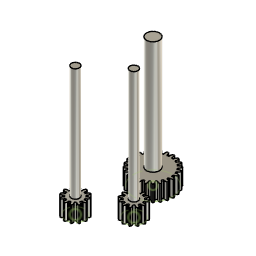
axle with gears v1 (Autodesk Fusion 360 design; units mm, degrees)
description: Spur Gear; Module: 2.000000; Num Teeth: 24; Pressure Angle: 20.000000; Backlash: 0.00 mm
description: Spur Gear; Module: 1.000000; Num Teeth: 24; Pressure Angle: 20.000000; Backlash: 0.00 mm
description: Spur Gear; Module: 0.500000; Num Teeth: 12; Pressure Angle: 20.000000; Backlash: 0.00 mm
description: Spur Gear; Module: 1.000000; Num Teeth: 12; Pressure Angle: 20.000000; Backlash: 0.00 mm
Autodesk Fusion 360 part; units mm, degrees
(part 1 of 7)
sketch "Sketch1" plane through (0, 0, 0) normal (0, 0, 1) x (1, 0, 0)
sketch "Sketch1 (2)" plane through (0, 0, 0) normal (0, 0, 1) x (1, 0, 0) in component "Spur Gear (24 teeth)"
  circle A0 centre (0, 0) radius 21.5492
extrude "Extrude1" [suppressed] in component "Spur Gear (24 teeth)"
sketch "Sketch2" plane through (0, 0, 0) normal (0, 0, 1) x (1, 0, 0) in component "Spur Gear (24 teeth)"
  spline S0 degree 5 poles (22.4799, -1.8102) (22.4899, -1.8111) (22.5101, -1.8124) (22.5404, -1.8137) (22.5808, -1.814) (22.6313, -1.8123) (22.6819, -1.8093) (22.7326, -1.8054) (22.7832, -1.801) (22.8339, -1.7962) (22.8846, -1.7911) (22.9353, -1.7856) (22.986, -1.7795) (23.0367, -1.7727) (23.0874, -1.7652) (23.1381, -1.7571) (23.1889, -1.7484) (23.2396, -1.7393) (23.2903, -1.7297) (23.341, -1.7198) (23.3916, -1.7095) (23.4423, -1.6988) (23.493, -1.6877) (23.5436, -1.6762) (23.5943, -1.6642) (23.6449, -1.6518) (23.6955, -1.6391) (23.7461, -1.6259) (23.7966, -1.6124) (23.8472, -1.5986) (23.8977, -1.5844) (23.9482, -1.5699) (23.9987, -1.555) (24.0491, -1.5398) (24.0996, -1.5242) (24.15, -1.5083) (24.2004, -1.4921) (24.2507, -1.4756) (24.301, -1.4587) (24.3513, -1.4415) (24.4016, -1.424) (24.4518, -1.4062) (24.502, -1.3881) (24.5522, -1.3697) (24.6024, -1.351) (24.6525, -1.3321) (24.7025, -1.3128) (24.7526, -1.2932) (24.8026, -1.2733) (24.8525, -1.2532) (24.9025, -1.2327) (24.9523, -1.212) (25.0022, -1.191) (25.052, -1.1697) (25.1018, -1.1482) (25.1515, -1.1264) (25.2012, -1.1043) (25.2509, -1.0819) (25.3005, -1.0593) (25.35, -1.0364) (25.3995, -1.0133) (25.449, -0.9898) (25.4985, -0.9662) (25.5478, -0.9422) (25.5972, -0.9181) (25.6465, -0.8936) (25.6957, -0.8689) (25.7449, -0.844) (25.7941, -0.8188) (25.8432, -0.7933) (25.8922, -0.7676) (25.9314, -0.7469) (25.9608, -0.7312) (25.9804, -0.7207) (25.9902, -0.7155) knots 0 0 0 0 0 0 0.01428571 0.02857143 0.04285714 0.05714286 0.07142857 0.08571429 0.1 0.11428571 0.12857143 0.14285714 0.15714286 0.17142857 0.18571429 0.2 0.21428571 0.22857143 0.24285714 0.25714286 0.27142857 0.28571429 0.3 0.31428571 0.32857143 0.34285714 0.35714286 0.37142857 0.38571429 0.4 0.41428571 0.42857143 0.44285714 0.45714286 0.47142857 0.48571429 0.5 0.51428571 0.52857143 0.54285714 0.55714286 0.57142857 0.58571429 0.6 0.61428571 0.62857143 0.64285714 0.65714286 0.67142857 0.68571429 0.7 0.71428571 0.72857143 0.74285714 0.75714286 0.77142857 0.78571429 0.8 0.81428571 0.82857143 0.84285714 0.85714286 0.87142857 0.88571429 0.9 0.91428571 0.92857143 0.94285714 0.95714286 0.97142857 0.98571429 1 1 1 1 1 1
  spline S1 degree 5 poles (22.4799, 1.8102) (22.4899, 1.8111) (22.5101, 1.8124) (22.5404, 1.8137) (22.5808, 1.814) (22.6313, 1.8123) (22.6819, 1.8093) (22.7326, 1.8054) (22.7832, 1.801) (22.8339, 1.7962) (22.8846, 1.7911) (22.9353, 1.7856) (22.986, 1.7795) (23.0367, 1.7727) (23.0874, 1.7652) (23.1381, 1.7571) (23.1889, 1.7484) (23.2396, 1.7393) (23.2903, 1.7297) (23.341, 1.7198) (23.3916, 1.7095) (23.4423, 1.6988) (23.493, 1.6877) (23.5436, 1.6762) (23.5943, 1.6642) (23.6449, 1.6518) (23.6955, 1.6391) (23.7461, 1.6259) (23.7966, 1.6124) (23.8472, 1.5986) (23.8977, 1.5844) (23.9482, 1.5699) (23.9987, 1.555) (24.0491, 1.5398) (24.0996, 1.5242) (24.15, 1.5083) (24.2004, 1.4921) (24.2507, 1.4756) (24.301, 1.4587) (24.3513, 1.4415) (24.4016, 1.424) (24.4518, 1.4062) (24.502, 1.3881) (24.5522, 1.3697) (24.6024, 1.351) (24.6525, 1.3321) (24.7025, 1.3128) (24.7526, 1.2932) (24.8026, 1.2733) (24.8525, 1.2532) (24.9025, 1.2327) (24.9523, 1.212) (25.0022, 1.191) (25.052, 1.1697) (25.1018, 1.1482) (25.1515, 1.1264) (25.2012, 1.1043) (25.2509, 1.0819) (25.3005, 1.0593) (25.35, 1.0364) (25.3995, 1.0133) (25.449, 0.9898) (25.4985, 0.9662) (25.5478, 0.9422) (25.5972, 0.9181) (25.6465, 0.8936) (25.6957, 0.8689) (25.7449, 0.844) (25.7941, 0.8188) (25.8432, 0.7933) (25.8922, 0.7676) (25.9314, 0.7469) (25.9608, 0.7312) (25.9804, 0.7207) (25.9902, 0.7155) knots 0 0 0 0 0 0 0.01428571 0.02857143 0.04285714 0.05714286 0.07142857 0.08571429 0.1 0.11428571 0.12857143 0.14285714 0.15714286 0.17142857 0.18571429 0.2 0.21428571 0.22857143 0.24285714 0.25714286 0.27142857 0.28571429 0.3 0.31428571 0.32857143 0.34285714 0.35714286 0.37142857 0.38571429 0.4 0.41428571 0.42857143 0.44285714 0.45714286 0.47142857 0.48571429 0.5 0.51428571 0.52857143 0.54285714 0.55714286 0.57142857 0.58571429 0.6 0.61428571 0.62857143 0.64285714 0.65714286 0.67142857 0.68571429 0.7 0.71428571 0.72857143 0.74285714 0.75714286 0.77142857 0.78571429 0.8 0.81428571 0.82857143 0.84285714 0.85714286 0.87142857 0.88571429 0.9 0.91428571 0.92857143 0.94285714 0.95714286 0.97142857 0.98571429 1 1 1 1 1 1
  arc A0 (25.9902, -0.7155) -> (25.9902, 0.7155) centre (0, 0) ccw
  line L0 (21.4697, -1.7297) -> (22.4799, -1.8102)
  line L1 (21.4697, 1.7297) -> (22.4799, 1.8102)
  line L2 (21.4697, -1.7297) -> (21.4697, 1.7297)
  point P0 (22.7272, -1.8057)
  point P1 (22.9762, -1.7806)
  point P2 (23.2261, -1.7416)
  point P3 (23.4768, -1.6912)
  point P4 (23.7279, -1.6306)
  point P5 (23.9793, -1.5607)
  point P6 (24.231, -1.482)
  point P7 (24.4828, -1.395)
  point P8 (24.7346, -1.3002)
  point P9 (24.9863, -1.1976)
  point P10 (25.2378, -1.0877)
  point P11 (25.489, -0.9706)
  point P12 (25.7398, -0.8465)
  point P13 (22.7272, 1.8057)
  point P14 (22.9762, 1.7806)
  point P15 (23.2261, 1.7416)
  point P16 (23.4768, 1.6912)
  point P17 (23.7279, 1.6306)
  point P18 (23.9793, 1.5607)
  point P19 (24.231, 1.482)
  point P20 (24.4828, 1.395)
  point P21 (24.7346, 1.3002)
  point P22 (24.9863, 1.1976)
  point P23 (25.2378, 1.0877)
  point P24 (25.489, 0.9706)
  point P25 (25.7398, 0.8465)
extrude "Extrude2" [suppressed] in component "Spur Gear (24 teeth)"
pattern_circular "C-Pattern1" [suppressed] in component "Spur Gear (24 teeth)"
sketch "Sketch3" plane through (0, 0, 0) normal (0, 0, 1) x (1, 0, 0) in component "Spur Gear (24 teeth)"
  circle A0 centre (0, 0) radius 24 construction
sketch "Sketch1 (3)" plane through (0, 0, 0) normal (0, 0, 1) x (1, 0, 0) in component "Spur Gear (24 teeth) (1)"
  circle A0 centre (0, 0) radius 10.7492
extrude "Extrude1'" add sketch "Sketch1 (3)" along normal blind 10 makes body 1 in component "Spur Gear (24 teeth) (1)"
sketch "Sketch2 (2)" plane through (0, 0, 0) normal (0, 0, 1) x (1, 0, 0) in component "Spur Gear (24 teeth) (1)"
  spline S0 degree 5 poles (11.2399, -0.9051) (11.2449, -0.9055) (11.255, -0.9062) (11.27, -0.9068) (11.2901, -0.907) (11.3152, -0.9062) (11.3404, -0.9047) (11.3655, -0.9028) (11.3907, -0.9006) (11.416, -0.8982) (11.4412, -0.8957) (11.4664, -0.8929) (11.4917, -0.8899) (11.5169, -0.8866) (11.5422, -0.8828) (11.5674, -0.8788) (11.5927, -0.8745) (11.6179, -0.87) (11.6432, -0.8652) (11.6685, -0.8603) (11.6937, -0.8552) (11.719, -0.8499) (11.7443, -0.8443) (11.7695, -0.8386) (11.7948, -0.8327) (11.82, -0.8265) (11.8453, -0.8202) (11.8706, -0.8136) (11.8958, -0.8069) (11.921, -0.8) (11.9463, -0.7929) (11.9715, -0.7857) (11.9967, -0.7783) (12.0219, -0.7707) (12.0471, -0.7629) (12.0723, -0.755) (12.0975, -0.7469) (12.1227, -0.7387) (12.1479, -0.7302) (12.173, -0.7217) (12.1982, -0.7129) (12.2233, -0.7041) (12.2484, -0.695) (12.2735, -0.6858) (12.2986, -0.6765) (12.3237, -0.667) (12.3488, -0.6573) (12.3739, -0.6475) (12.3989, -0.6376) (12.424, -0.6275) (12.449, -0.6173) (12.474, -0.6069) (12.499, -0.5964) (12.5239, -0.5858) (12.5489, -0.575) (12.5738, -0.564) (12.5988, -0.553) (12.6237, -0.5418) (12.6486, -0.5304) (12.6735, -0.5189) (12.6983, -0.5073) (12.7232, -0.4956) (12.748, -0.4837) (12.7728, -0.4717) (12.7976, -0.4595) (12.8223, -0.4473) (12.8471, -0.4349) (12.8718, -0.4223) (12.8965, -0.4097) (12.9212, -0.3969) (12.9458, -0.384) (12.9655, -0.3735) (12.9803, -0.3657) (12.9902, -0.3604) (12.9951, -0.3577) knots 0 0 0 0 0 0 0.01428571 0.02857143 0.04285714 0.05714286 0.07142857 0.08571429 0.1 0.11428571 0.12857143 0.14285714 0.15714286 0.17142857 0.18571429 0.2 0.21428571 0.22857143 0.24285714 0.25714286 0.27142857 0.28571429 0.3 0.31428571 0.32857143 0.34285714 0.35714286 0.37142857 0.38571429 0.4 0.41428571 0.42857143 0.44285714 0.45714286 0.47142857 0.48571429 0.5 0.51428571 0.52857143 0.54285714 0.55714286 0.57142857 0.58571429 0.6 0.61428571 0.62857143 0.64285714 0.65714286 0.67142857 0.68571429 0.7 0.71428571 0.72857143 0.74285714 0.75714286 0.77142857 0.78571429 0.8 0.81428571 0.82857143 0.84285714 0.85714286 0.87142857 0.88571429 0.9 0.91428571 0.92857143 0.94285714 0.95714286 0.97142857 0.98571429 1 1 1 1 1 1
  spline S1 degree 5 poles (11.2399, 0.9051) (11.2449, 0.9055) (11.255, 0.9062) (11.27, 0.9068) (11.2901, 0.907) (11.3152, 0.9062) (11.3404, 0.9047) (11.3655, 0.9028) (11.3907, 0.9006) (11.416, 0.8982) (11.4412, 0.8957) (11.4664, 0.8929) (11.4917, 0.8899) (11.5169, 0.8866) (11.5422, 0.8828) (11.5674, 0.8788) (11.5927, 0.8745) (11.6179, 0.87) (11.6432, 0.8652) (11.6685, 0.8603) (11.6937, 0.8552) (11.719, 0.8499) (11.7443, 0.8443) (11.7695, 0.8386) (11.7948, 0.8327) (11.82, 0.8265) (11.8453, 0.8202) (11.8706, 0.8136) (11.8958, 0.8069) (11.921, 0.8) (11.9463, 0.7929) (11.9715, 0.7857) (11.9967, 0.7783) (12.0219, 0.7707) (12.0471, 0.7629) (12.0723, 0.755) (12.0975, 0.7469) (12.1227, 0.7387) (12.1479, 0.7302) (12.173, 0.7217) (12.1982, 0.7129) (12.2233, 0.7041) (12.2484, 0.695) (12.2735, 0.6858) (12.2986, 0.6765) (12.3237, 0.667) (12.3488, 0.6573) (12.3739, 0.6475) (12.3989, 0.6376) (12.424, 0.6275) (12.449, 0.6173) (12.474, 0.6069) (12.499, 0.5964) (12.5239, 0.5858) (12.5489, 0.575) (12.5738, 0.564) (12.5988, 0.553) (12.6237, 0.5418) (12.6486, 0.5304) (12.6735, 0.5189) (12.6983, 0.5073) (12.7232, 0.4956) (12.748, 0.4837) (12.7728, 0.4717) (12.7976, 0.4595) (12.8223, 0.4473) (12.8471, 0.4349) (12.8718, 0.4223) (12.8965, 0.4097) (12.9212, 0.3969) (12.9458, 0.384) (12.9655, 0.3735) (12.9803, 0.3657) (12.9902, 0.3604) (12.9951, 0.3577) knots 0 0 0 0 0 0 0.01428571 0.02857143 0.04285714 0.05714286 0.07142857 0.08571429 0.1 0.11428571 0.12857143 0.14285714 0.15714286 0.17142857 0.18571429 0.2 0.21428571 0.22857143 0.24285714 0.25714286 0.27142857 0.28571429 0.3 0.31428571 0.32857143 0.34285714 0.35714286 0.37142857 0.38571429 0.4 0.41428571 0.42857143 0.44285714 0.45714286 0.47142857 0.48571429 0.5 0.51428571 0.52857143 0.54285714 0.55714286 0.57142857 0.58571429 0.6 0.61428571 0.62857143 0.64285714 0.65714286 0.67142857 0.68571429 0.7 0.71428571 0.72857143 0.74285714 0.75714286 0.77142857 0.78571429 0.8 0.81428571 0.82857143 0.84285714 0.85714286 0.87142857 0.88571429 0.9 0.91428571 0.92857143 0.94285714 0.95714286 0.97142857 0.98571429 1 1 1 1 1 1
  arc A0 (12.9951, -0.3577) -> (12.9951, 0.3577) centre (0, 0) ccw
  line L0 (10.7045, -0.8628) -> (11.2399, -0.9051)
  line L1 (10.7045, 0.8628) -> (11.2399, 0.9051)
  line L2 (10.7045, -0.8628) -> (10.7045, 0.8628)
  point P0 (11.3636, -0.9028)
  point P1 (11.4881, -0.8903)
  point P2 (11.6131, -0.8708)
  point P3 (11.7384, -0.8456)
  point P4 (11.8639, -0.8153)
  point P5 (11.9897, -0.7803)
  point P6 (12.1155, -0.741)
  point P7 (12.2414, -0.6975)
  point P8 (12.3673, -0.6501)
  point P9 (12.4932, -0.5988)
  point P10 (12.6189, -0.5439)
  point P11 (12.7445, -0.4853)
  point P12 (12.8699, -0.4232)
  point P13 (11.3636, 0.9028)
  point P14 (11.4881, 0.8903)
  point P15 (11.6131, 0.8708)
  point P16 (11.7384, 0.8456)
  point P17 (11.8639, 0.8153)
  point P18 (11.9897, 0.7803)
  point P19 (12.1155, 0.741)
  point P20 (12.2414, 0.6975)
  point P21 (12.3673, 0.6501)
  point P22 (12.4932, 0.5988)
  point P23 (12.6189, 0.5439)
  point P24 (12.7445, 0.4853)
  point P25 (12.8699, 0.4232)
extrude "Extrude2'" add sketch "Sketch2 (2)" along normal blind 10 bodies 1 in component "Spur Gear (24 teeth) (1)"
pattern_circular "C-Pattern1'" count 24 over 360 about axis through (0, 0, 0) along (0, 0, 1) of "Extrude2'" in component "Spur Gear (24 teeth) (1)"
sketch "Sketch3 (2)" plane through (0, 0, 0) normal (0, 0, 1) x (1, 0, 0) in component "Spur Gear (24 teeth) (1)"
  circle A0 centre (0, 0) radius 12 construction
sketch "Sketch2 (3)" plane through (0, 0, 0) normal (0, 0, -1) x (1, 0, 0)
  arc A0 (10.1259, 3.6073) -> (9.7108, 4.6093) centre (0, 0) ccw
  line L0 (9.7108, 4.6093) -> (10.1866, 4.8361)
  spline S0 degree 5 poles (10.1866, 4.8361) (10.1912, 4.8383) (10.2002, 4.8427) (10.2135, 4.8497) (10.231, 4.8596) (10.2523, 4.8728) (10.2734, 4.8867) (10.2942, 4.901) (10.315, 4.9155) (10.3356, 4.9301) (10.3562, 4.9449) (10.3767, 4.9599) (10.397, 4.9751) (10.4172, 4.9907) (10.4372, 5.0065) (10.4571, 5.0226) (10.4768, 5.039) (10.4964, 5.0555) (10.5159, 5.0723) (10.5353, 5.0892) (10.5547, 5.1063) (10.5739, 5.1235) (10.593, 5.1409) (10.612, 5.1585) (10.6309, 5.1763) (10.6497, 5.1942) (10.6684, 5.2124) (10.687, 5.2307) (10.7055, 5.2491) (10.7239, 5.2677) (10.7422, 5.2864) (10.7605, 5.3053) (10.7786, 5.3243) (10.7966, 5.3435) (10.8146, 5.3628) (10.8324, 5.3823) (10.8502, 5.4019) (10.8679, 5.4216) (10.8855, 5.4415) (10.903, 5.4615) (10.9204, 5.4817) (10.9377, 5.5019) (10.955, 5.5223) (10.9721, 5.5428) (10.9892, 5.5635) (11.0062, 5.5842) (11.023, 5.6051) (11.0399, 5.6261) (11.0566, 5.6473) (11.0732, 5.6685) (11.0898, 5.6899) (11.1062, 5.7114) (11.1226, 5.733) (11.1389, 5.7547) (11.1552, 5.7765) (11.1713, 5.7985) (11.1873, 5.8205) (11.2033, 5.8427) (11.2192, 5.8649) (11.235, 5.8873) (11.2507, 5.9098) (11.2664, 5.9324) (11.2819, 5.9551) (11.2974, 5.9779) (11.3128, 6.0008) (11.3281, 6.0238) (11.3433, 6.0469) (11.3585, 6.0701) (11.3735, 6.0935) (11.3885, 6.1169) (11.4034, 6.1404) (11.4153, 6.1593) (11.4241, 6.1735) (11.43, 6.183) (11.4329, 6.1877) knots 0 0 0 0 0 0 0.01428571 0.02857143 0.04285714 0.05714286 0.07142857 0.08571429 0.1 0.11428571 0.12857143 0.14285714 0.15714286 0.17142857 0.18571429 0.2 0.21428571 0.22857143 0.24285714 0.25714286 0.27142857 0.28571429 0.3 0.31428571 0.32857143 0.34285714 0.35714286 0.37142857 0.38571429 0.4 0.41428571 0.42857143 0.44285714 0.45714286 0.47142857 0.48571429 0.5 0.51428571 0.52857143 0.54285714 0.55714286 0.57142857 0.58571429 0.6 0.61428571 0.62857143 0.64285714 0.65714286 0.67142857 0.68571429 0.7 0.71428571 0.72857143 0.74285714 0.75714286 0.77142857 0.78571429 0.8 0.81428571 0.82857143 0.84285714 0.85714286 0.87142857 0.88571429 0.9 0.91428571 0.92857143 0.94285714 0.95714286 0.97142857 0.98571429 1 1 1 1 1 1
  arc A1 (11.4329, 6.1877) -> (11.0752, 6.8073) centre (0, 0) ccw
  spline S1 degree 5 poles (9.2815, 6.4038) (9.2856, 6.4067) (9.294, 6.4123) (9.3067, 6.4203) (9.324, 6.4305) (9.3462, 6.4424) (9.3687, 6.4537) (9.3915, 6.4646) (9.4144, 6.4753) (9.4374, 6.4859) (9.4605, 6.4963) (9.4837, 6.5065) (9.5071, 6.5165) (9.5307, 6.5262) (9.5544, 6.5356) (9.5783, 6.5448) (9.6023, 6.5537) (9.6264, 6.5624) (9.6507, 6.5709) (9.675, 6.5793) (9.6995, 6.5875) (9.724, 6.5955) (9.7487, 6.6034) (9.7734, 6.611) (9.7983, 6.6185) (9.8232, 6.6258) (9.8483, 6.6329) (9.8734, 6.6399) (9.8986, 6.6467) (9.9239, 6.6533) (9.9493, 6.6598) (9.9748, 6.6662) (10.0003, 6.6724) (10.0259, 6.6784) (10.0516, 6.6843) (10.0774, 6.69) (10.1033, 6.6956) (10.1292, 6.701) (10.1552, 6.7063) (10.1813, 6.7115) (10.2074, 6.7165) (10.2337, 6.7214) (10.2599, 6.7261) (10.2863, 6.7307) (10.3127, 6.7352) (10.3392, 6.7395) (10.3657, 6.7437) (10.3923, 6.7477) (10.419, 6.7516) (10.4457, 6.7554) (10.4725, 6.7591) (10.4993, 6.7626) (10.5262, 6.766) (10.5532, 6.7693) (10.5802, 6.7724) (10.6073, 6.7754) (10.6344, 6.7783) (10.6616, 6.781) (10.6888, 6.7836) (10.7161, 6.7861) (10.7434, 6.7885) (10.7708, 6.7908) (10.7982, 6.7929) (10.8257, 6.7949) (10.8532, 6.7967) (10.8808, 6.7985) (10.9085, 6.8001) (10.9361, 6.8016) (10.9638, 6.803) (10.9916, 6.8043) (11.0194, 6.8054) (11.0417, 6.8063) (11.0585, 6.8068) (11.0696, 6.8072) (11.0752, 6.8073) knots 0 0 0 0 0 0 0.01428571 0.02857143 0.04285714 0.05714286 0.07142857 0.08571429 0.1 0.11428571 0.12857143 0.14285714 0.15714286 0.17142857 0.18571429 0.2 0.21428571 0.22857143 0.24285714 0.25714286 0.27142857 0.28571429 0.3 0.31428571 0.32857143 0.34285714 0.35714286 0.37142857 0.38571429 0.4 0.41428571 0.42857143 0.44285714 0.45714286 0.47142857 0.48571429 0.5 0.51428571 0.52857143 0.54285714 0.55714286 0.57142857 0.58571429 0.6 0.61428571 0.62857143 0.64285714 0.65714286 0.67142857 0.68571429 0.7 0.71428571 0.72857143 0.74285714 0.75714286 0.77142857 0.78571429 0.8 0.81428571 0.82857143 0.84285714 0.85714286 0.87142857 0.88571429 0.9 0.91428571 0.92857143 0.94285714 0.95714286 0.97142857 0.98571429 1 1 1 1 1 1
  line L1 (9.2815, 6.4038) -> (8.8472, 6.1051)
  arc A2 (8.8472, 6.1051) -> (8.1869, 6.9656) centre (0, 0) ccw
  line L2 (8.1869, 6.9656) -> (8.5878, 7.3078)
  spline S2 degree 5 poles (8.5878, 7.3078) (8.5917, 7.3111) (8.5992, 7.3177) (8.6103, 7.3279) (8.6246, 7.342) (8.6418, 7.3603) (8.6586, 7.3791) (8.675, 7.3983) (8.6913, 7.4177) (8.7074, 7.4372) (8.7235, 7.4568) (8.7394, 7.4766) (8.7551, 7.4966) (8.7706, 7.5168) (8.7858, 7.5373) (8.8008, 7.558) (8.8156, 7.5789) (8.8303, 7.6) (8.8448, 7.6212) (8.8592, 7.6425) (8.8734, 7.664) (8.8875, 7.6856) (8.9015, 7.7074) (8.9153, 7.7293) (8.929, 7.7514) (8.9425, 7.7736) (8.9558, 7.796) (8.9691, 7.8184) (8.9822, 7.841) (8.9951, 7.8638) (9.008, 7.8866) (9.0207, 7.9096) (9.0333, 7.9326) (9.0457, 7.9558) (9.0581, 7.9791) (9.0703, 8.0025) (9.0824, 8.0261) (9.0943, 8.0497) (9.1062, 8.0735) (9.1179, 8.0973) (9.1295, 8.1213) (9.141, 8.1453) (9.1524, 8.1695) (9.1637, 8.1938) (9.1748, 8.2181) (9.1858, 8.2426) (9.1967, 8.2671) (9.2075, 8.2918) (9.2182, 8.3165) (9.2288, 8.3413) (9.2392, 8.3663) (9.2496, 8.3913) (9.2598, 8.4164) (9.27, 8.4416) (9.28, 8.4669) (9.2899, 8.4922) (9.2997, 8.5177) (9.3094, 8.5432) (9.319, 8.5688) (9.3284, 8.5945) (9.3378, 8.6203) (9.347, 8.6462) (9.3562, 8.6722) (9.3652, 8.6982) (9.3742, 8.7243) (9.383, 8.7505) (9.3917, 8.7768) (9.4004, 8.8031) (9.4089, 8.8295) (9.4173, 8.856) (9.4256, 8.8826) (9.4321, 8.9039) (9.437, 8.9199) (9.4403, 8.9306) (9.4419, 8.936) knots 0 0 0 0 0 0 0.01428571 0.02857143 0.04285714 0.05714286 0.07142857 0.08571429 0.1 0.11428571 0.12857143 0.14285714 0.15714286 0.17142857 0.18571429 0.2 0.21428571 0.22857143 0.24285714 0.25714286 0.27142857 0.28571429 0.3 0.31428571 0.32857143 0.34285714 0.35714286 0.37142857 0.38571429 0.4 0.41428571 0.42857143 0.44285714 0.45714286 0.47142857 0.48571429 0.5 0.51428571 0.52857143 0.54285714 0.55714286 0.57142857 0.58571429 0.6 0.61428571 0.62857143 0.64285714 0.65714286 0.67142857 0.68571429 0.7 0.71428571 0.72857143 0.74285714 0.75714286 0.77142857 0.78571429 0.8 0.81428571 0.82857143 0.84285714 0.85714286 0.87142857 0.88571429 0.9 0.91428571 0.92857143 0.94285714 0.95714286 0.97142857 0.98571429 1 1 1 1 1 1
  arc A3 (9.4419, 8.936) -> (8.936, 9.4419) centre (0, 0) ccw
  spline S3 degree 5 poles (7.3078, 8.5878) (7.3111, 8.5917) (7.3177, 8.5992) (7.3279, 8.6103) (7.342, 8.6246) (7.3603, 8.6418) (7.3791, 8.6586) (7.3983, 8.675) (7.4177, 8.6913) (7.4372, 8.7074) (7.4568, 8.7235) (7.4766, 8.7394) (7.4966, 8.7551) (7.5168, 8.7706) (7.5373, 8.7858) (7.558, 8.8008) (7.5789, 8.8156) (7.6, 8.8303) (7.6212, 8.8448) (7.6425, 8.8592) (7.664, 8.8734) (7.6856, 8.8875) (7.7074, 8.9015) (7.7293, 8.9153) (7.7514, 8.929) (7.7736, 8.9425) (7.796, 8.9558) (7.8184, 8.9691) (7.841, 8.9822) (7.8638, 8.9951) (7.8866, 9.008) (7.9096, 9.0207) (7.9326, 9.0333) (7.9558, 9.0457) (7.9791, 9.0581) (8.0025, 9.0703) (8.0261, 9.0824) (8.0497, 9.0943) (8.0735, 9.1062) (8.0973, 9.1179) (8.1213, 9.1295) (8.1453, 9.141) (8.1695, 9.1524) (8.1938, 9.1637) (8.2181, 9.1748) (8.2426, 9.1858) (8.2671, 9.1967) (8.2918, 9.2075) (8.3165, 9.2182) (8.3413, 9.2288) (8.3663, 9.2392) (8.3913, 9.2496) (8.4164, 9.2598) (8.4416, 9.27) (8.4669, 9.28) (8.4922, 9.2899) (8.5177, 9.2997) (8.5432, 9.3094) (8.5688, 9.319) (8.5945, 9.3284) (8.6203, 9.3378) (8.6462, 9.347) (8.6722, 9.3562) (8.6982, 9.3652) (8.7243, 9.3742) (8.7505, 9.383) (8.7768, 9.3917) (8.8031, 9.4004) (8.8295, 9.4089) (8.856, 9.4173) (8.8826, 9.4256) (8.9039, 9.4321) (8.9199, 9.437) (8.9306, 9.4403) (8.936, 9.4419) knots 0 0 0 0 0 0 0.01428571 0.02857143 0.04285714 0.05714286 0.07142857 0.08571429 0.1 0.11428571 0.12857143 0.14285714 0.15714286 0.17142857 0.18571429 0.2 0.21428571 0.22857143 0.24285714 0.25714286 0.27142857 0.28571429 0.3 0.31428571 0.32857143 0.34285714 0.35714286 0.37142857 0.38571429 0.4 0.41428571 0.42857143 0.44285714 0.45714286 0.47142857 0.48571429 0.5 0.51428571 0.52857143 0.54285714 0.55714286 0.57142857 0.58571429 0.6 0.61428571 0.62857143 0.64285714 0.65714286 0.67142857 0.68571429 0.7 0.71428571 0.72857143 0.74285714 0.75714286 0.77142857 0.78571429 0.8 0.81428571 0.82857143 0.84285714 0.85714286 0.87142857 0.88571429 0.9 0.91428571 0.92857143 0.94285714 0.95714286 0.97142857 0.98571429 1 1 1 1 1 1
  line L3 (7.3078, 8.5878) -> (6.9656, 8.1869)
  arc A4 (6.9656, 8.1869) -> (6.1051, 8.8472) centre (0, 0) ccw
  line L4 (6.1051, 8.8472) -> (6.4038, 9.2815)
  spline S4 degree 5 poles (6.4038, 9.2815) (6.4067, 9.2856) (6.4123, 9.294) (6.4203, 9.3067) (6.4305, 9.324) (6.4424, 9.3462) (6.4537, 9.3687) (6.4646, 9.3915) (6.4753, 9.4144) (6.4859, 9.4374) (6.4963, 9.4605) (6.5065, 9.4837) (6.5165, 9.5071) (6.5262, 9.5307) (6.5356, 9.5544) (6.5448, 9.5783) (6.5537, 9.6023) (6.5624, 9.6264) (6.5709, 9.6507) (6.5793, 9.675) (6.5875, 9.6995) (6.5955, 9.724) (6.6034, 9.7487) (6.611, 9.7734) (6.6185, 9.7983) (6.6258, 9.8232) (6.6329, 9.8483) (6.6399, 9.8734) (6.6467, 9.8986) (6.6533, 9.9239) (6.6598, 9.9493) (6.6662, 9.9748) (6.6724, 10.0003) (6.6784, 10.0259) (6.6843, 10.0516) (6.69, 10.0774) (6.6956, 10.1033) (6.701, 10.1292) (6.7063, 10.1552) (6.7115, 10.1813) (6.7165, 10.2074) (6.7214, 10.2337) (6.7261, 10.2599) (6.7307, 10.2863) (6.7352, 10.3127) (6.7395, 10.3392) (6.7437, 10.3657) (6.7477, 10.3923) (6.7516, 10.419) (6.7554, 10.4457) (6.7591, 10.4725) (6.7626, 10.4993) (6.766, 10.5262) (6.7693, 10.5532) (6.7724, 10.5802) (6.7754, 10.6073) (6.7783, 10.6344) (6.781, 10.6616) (6.7836, 10.6888) (6.7861, 10.7161) (6.7885, 10.7434) (6.7908, 10.7708) (6.7929, 10.7982) (6.7949, 10.8257) (6.7967, 10.8532) (6.7985, 10.8808) (6.8001, 10.9085) (6.8016, 10.9361) (6.803, 10.9638) (6.8043, 10.9916) (6.8054, 11.0194) (6.8063, 11.0417) (6.8068, 11.0585) (6.8072, 11.0696) (6.8073, 11.0752) knots 0 0 0 0 0 0 0.01428571 0.02857143 0.04285714 0.05714286 0.07142857 0.08571429 0.1 0.11428571 0.12857143 0.14285714 0.15714286 0.17142857 0.18571429 0.2 0.21428571 0.22857143 0.24285714 0.25714286 0.27142857 0.28571429 0.3 0.31428571 0.32857143 0.34285714 0.35714286 0.37142857 0.38571429 0.4 0.41428571 0.42857143 0.44285714 0.45714286 0.47142857 0.48571429 0.5 0.51428571 0.52857143 0.54285714 0.55714286 0.57142857 0.58571429 0.6 0.61428571 0.62857143 0.64285714 0.65714286 0.67142857 0.68571429 0.7 0.71428571 0.72857143 0.74285714 0.75714286 0.77142857 0.78571429 0.8 0.81428571 0.82857143 0.84285714 0.85714286 0.87142857 0.88571429 0.9 0.91428571 0.92857143 0.94285714 0.95714286 0.97142857 0.98571429 1 1 1 1 1 1
  arc A5 (6.8073, 11.0752) -> (6.1877, 11.4329) centre (0, 0) ccw
  spline S5 degree 5 poles (4.8361, 10.1866) (4.8383, 10.1912) (4.8427, 10.2002) (4.8497, 10.2135) (4.8596, 10.231) (4.8728, 10.2523) (4.8867, 10.2734) (4.901, 10.2942) (4.9155, 10.315) (4.9301, 10.3356) (4.9449, 10.3562) (4.9599, 10.3767) (4.9751, 10.397) (4.9907, 10.4172) (5.0065, 10.4372) (5.0226, 10.4571) (5.039, 10.4768) (5.0555, 10.4964) (5.0723, 10.5159) (5.0892, 10.5353) (5.1063, 10.5547) (5.1235, 10.5739) (5.1409, 10.593) (5.1585, 10.612) (5.1763, 10.6309) (5.1942, 10.6497) (5.2124, 10.6684) (5.2307, 10.687) (5.2491, 10.7055) (5.2677, 10.7239) (5.2864, 10.7422) (5.3053, 10.7605) (5.3243, 10.7786) (5.3435, 10.7966) (5.3628, 10.8146) (5.3823, 10.8324) (5.4019, 10.8502) (5.4216, 10.8679) (5.4415, 10.8855) (5.4615, 10.903) (5.4817, 10.9204) (5.5019, 10.9377) (5.5223, 10.955) (5.5428, 10.9721) (5.5635, 10.9892) (5.5842, 11.0062) (5.6051, 11.023) (5.6261, 11.0399) (5.6473, 11.0566) (5.6685, 11.0732) (5.6899, 11.0898) (5.7114, 11.1062) (5.733, 11.1226) (5.7547, 11.1389) (5.7765, 11.1552) (5.7985, 11.1713) (5.8205, 11.1873) (5.8427, 11.2033) (5.8649, 11.2192) (5.8873, 11.235) (5.9098, 11.2507) (5.9324, 11.2664) (5.9551, 11.2819) (5.9779, 11.2974) (6.0008, 11.3128) (6.0238, 11.3281) (6.0469, 11.3433) (6.0701, 11.3585) (6.0935, 11.3735) (6.1169, 11.3885) (6.1404, 11.4034) (6.1593, 11.4153) (6.1735, 11.4241) (6.183, 11.43) (6.1877, 11.4329) knots 0 0 0 0 0 0 0.01428571 0.02857143 0.04285714 0.05714286 0.07142857 0.08571429 0.1 0.11428571 0.12857143 0.14285714 0.15714286 0.17142857 0.18571429 0.2 0.21428571 0.22857143 0.24285714 0.25714286 0.27142857 0.28571429 0.3 0.31428571 0.32857143 0.34285714 0.35714286 0.37142857 0.38571429 0.4 0.41428571 0.42857143 0.44285714 0.45714286 0.47142857 0.48571429 0.5 0.51428571 0.52857143 0.54285714 0.55714286 0.57142857 0.58571429 0.6 0.61428571 0.62857143 0.64285714 0.65714286 0.67142857 0.68571429 0.7 0.71428571 0.72857143 0.74285714 0.75714286 0.77142857 0.78571429 0.8 0.81428571 0.82857143 0.84285714 0.85714286 0.87142857 0.88571429 0.9 0.91428571 0.92857143 0.94285714 0.95714286 0.97142857 0.98571429 1 1 1 1 1 1
  line L5 (4.8361, 10.1866) -> (4.6093, 9.7108)
  arc A6 (4.6093, 9.7108) -> (3.6073, 10.1259) centre (0, 0) ccw
  line L6 (3.6073, 10.1259) -> (3.7834, 10.6227)
  spline S6 degree 5 poles (3.7834, 10.6227) (3.7851, 10.6274) (3.7883, 10.6369) (3.7928, 10.6513) (3.7981, 10.6706) (3.8039, 10.6951) (3.809, 10.7198) (3.8136, 10.7446) (3.818, 10.7695) (3.8223, 10.7945) (3.8264, 10.8195) (3.8302, 10.8446) (3.8339, 10.8698) (3.8371, 10.895) (3.8401, 10.9204) (3.8427, 10.9458) (3.8451, 10.9713) (3.8473, 10.9969) (3.8492, 11.0225) (3.851, 11.0482) (3.8526, 11.0739) (3.854, 11.0997) (3.8552, 11.1256) (3.8562, 11.1514) (3.857, 11.1774) (3.8576, 11.2034) (3.858, 11.2294) (3.8582, 11.2555) (3.8583, 11.2816) (3.8581, 11.3078) (3.8578, 11.334) (3.8574, 11.3602) (3.8567, 11.3865) (3.8559, 11.4128) (3.855, 11.4392) (3.8538, 11.4656) (3.8525, 11.492) (3.8511, 11.5184) (3.8495, 11.5449) (3.8477, 11.5714) (3.8458, 11.598) (3.8437, 11.6246) (3.8415, 11.6512) (3.8391, 11.6778) (3.8365, 11.7045) (3.8339, 11.7312) (3.831, 11.7579) (3.8281, 11.7846) (3.825, 11.8114) (3.8217, 11.8382) (3.8183, 11.865) (3.8147, 11.8919) (3.8111, 11.9187) (3.8072, 11.9456) (3.8033, 11.9725) (3.7992, 11.9994) (3.7949, 12.0264) (3.7905, 12.0533) (3.786, 12.0803) (3.7814, 12.1073) (3.7766, 12.1343) (3.7717, 12.1614) (3.7666, 12.1884) (3.7614, 12.2155) (3.7561, 12.2426) (3.7507, 12.2696) (3.7451, 12.2968) (3.7394, 12.3239) (3.7336, 12.351) (3.7276, 12.3782) (3.7215, 12.4053) (3.7165, 12.4271) (3.7127, 12.4434) (3.7102, 12.4543) (3.7089, 12.4597) knots 0 0 0 0 0 0 0.01428571 0.02857143 0.04285714 0.05714286 0.07142857 0.08571429 0.1 0.11428571 0.12857143 0.14285714 0.15714286 0.17142857 0.18571429 0.2 0.21428571 0.22857143 0.24285714 0.25714286 0.27142857 0.28571429 0.3 0.31428571 0.32857143 0.34285714 0.35714286 0.37142857 0.38571429 0.4 0.41428571 0.42857143 0.44285714 0.45714286 0.47142857 0.48571429 0.5 0.51428571 0.52857143 0.54285714 0.55714286 0.57142857 0.58571429 0.6 0.61428571 0.62857143 0.64285714 0.65714286 0.67142857 0.68571429 0.7 0.71428571 0.72857143 0.74285714 0.75714286 0.77142857 0.78571429 0.8 0.81428571 0.82857143 0.84285714 0.85714286 0.87142857 0.88571429 0.9 0.91428571 0.92857143 0.94285714 0.95714286 0.97142857 0.98571429 1 1 1 1 1 1
  arc A7 (3.7089, 12.4597) -> (3.0178, 12.6449) centre (0, 0) ccw
  spline S7 degree 5 poles (2.0348, 11.0912) (2.0357, 11.0961) (2.0377, 11.106) (2.041, 11.1207) (2.046, 11.1401) (2.0533, 11.1642) (2.0612, 11.1881) (2.0696, 11.2119) (2.0783, 11.2357) (2.0871, 11.2594) (2.096, 11.2831) (2.1052, 11.3068) (2.1147, 11.3304) (2.1244, 11.3539) (2.1346, 11.3774) (2.145, 11.4007) (2.1557, 11.424) (2.1666, 11.4472) (2.1777, 11.4704) (2.189, 11.4935) (2.2005, 11.5166) (2.2122, 11.5397) (2.2241, 11.5626) (2.2361, 11.5855) (2.2484, 11.6084) (2.2609, 11.6312) (2.2736, 11.654) (2.2864, 11.6767) (2.2995, 11.6993) (2.3126, 11.7219) (2.326, 11.7444) (2.3395, 11.7669) (2.3532, 11.7894) (2.3671, 11.8118) (2.3811, 11.8341) (2.3953, 11.8564) (2.4096, 11.8786) (2.4241, 11.9008) (2.4387, 11.9229) (2.4535, 11.945) (2.4685, 11.967) (2.4836, 11.989) (2.4988, 12.011) (2.5142, 12.0328) (2.5297, 12.0547) (2.5454, 12.0764) (2.5612, 12.0982) (2.5771, 12.1198) (2.5932, 12.1415) (2.6094, 12.163) (2.6258, 12.1846) (2.6423, 12.206) (2.6589, 12.2274) (2.6756, 12.2488) (2.6925, 12.2701) (2.7095, 12.2914) (2.7267, 12.3126) (2.744, 12.3338) (2.7614, 12.3549) (2.7789, 12.3759) (2.7965, 12.3969) (2.8143, 12.4179) (2.8322, 12.4388) (2.8502, 12.4596) (2.8684, 12.4804) (2.8866, 12.5012) (2.905, 12.5219) (2.9235, 12.5425) (2.9421, 12.5631) (2.9609, 12.5836) (2.9797, 12.6041) (2.9949, 12.6204) (3.0064, 12.6327) (3.014, 12.6408) (3.0178, 12.6449) knots 0 0 0 0 0 0 0.01428571 0.02857143 0.04285714 0.05714286 0.07142857 0.08571429 0.1 0.11428571 0.12857143 0.14285714 0.15714286 0.17142857 0.18571429 0.2 0.21428571 0.22857143 0.24285714 0.25714286 0.27142857 0.28571429 0.3 0.31428571 0.32857143 0.34285714 0.35714286 0.37142857 0.38571429 0.4 0.41428571 0.42857143 0.44285714 0.45714286 0.47142857 0.48571429 0.5 0.51428571 0.52857143 0.54285714 0.55714286 0.57142857 0.58571429 0.6 0.61428571 0.62857143 0.64285714 0.65714286 0.67142857 0.68571429 0.7 0.71428571 0.72857143 0.74285714 0.75714286 0.77142857 0.78571429 0.8 0.81428571 0.82857143 0.84285714 0.85714286 0.87142857 0.88571429 0.9 0.91428571 0.92857143 0.94285714 0.95714286 0.97142857 0.98571429 1 1 1 1 1 1
  line L7 (2.0348, 11.0912) -> (1.9389, 10.5729)
  arc A8 (1.9389, 10.5729) -> (0.8636, 10.7145) centre (0, 0) ccw
  line L8 (0.8636, 10.7145) -> (0.9051, 11.2399)
  spline S8 degree 5 poles (0.9051, 11.2399) (0.9055, 11.2449) (0.9062, 11.255) (0.9068, 11.27) (0.907, 11.2901) (0.9062, 11.3152) (0.9047, 11.3404) (0.9028, 11.3655) (0.9006, 11.3907) (0.8982, 11.416) (0.8957, 11.4412) (0.8929, 11.4664) (0.8899, 11.4917) (0.8866, 11.5169) (0.8828, 11.5422) (0.8788, 11.5674) (0.8745, 11.5927) (0.87, 11.6179) (0.8652, 11.6432) (0.8603, 11.6685) (0.8552, 11.6937) (0.8499, 11.719) (0.8443, 11.7443) (0.8386, 11.7695) (0.8327, 11.7948) (0.8265, 11.82) (0.8202, 11.8453) (0.8136, 11.8706) (0.8069, 11.8958) (0.8, 11.921) (0.7929, 11.9463) (0.7857, 11.9715) (0.7783, 11.9967) (0.7707, 12.0219) (0.7629, 12.0471) (0.755, 12.0723) (0.7469, 12.0975) (0.7387, 12.1227) (0.7302, 12.1479) (0.7217, 12.173) (0.7129, 12.1982) (0.7041, 12.2233) (0.695, 12.2484) (0.6858, 12.2735) (0.6765, 12.2986) (0.667, 12.3237) (0.6573, 12.3488) (0.6475, 12.3739) (0.6376, 12.3989) (0.6275, 12.424) (0.6173, 12.449) (0.6069, 12.474) (0.5964, 12.499) (0.5858, 12.5239) (0.575, 12.5489) (0.564, 12.5738) (0.553, 12.5988) (0.5418, 12.6237) (0.5304, 12.6486) (0.5189, 12.6735) (0.5073, 12.6983) (0.4956, 12.7232) (0.4837, 12.748) (0.4717, 12.7728) (0.4595, 12.7976) (0.4473, 12.8223) (0.4349, 12.8471) (0.4223, 12.8718) (0.4097, 12.8965) (0.3969, 12.9212) (0.384, 12.9458) (0.3735, 12.9655) (0.3657, 12.9803) (0.3604, 12.9902) (0.3577, 12.9951) knots 0 0 0 0 0 0 0.01428571 0.02857143 0.04285714 0.05714286 0.07142857 0.08571429 0.1 0.11428571 0.12857143 0.14285714 0.15714286 0.17142857 0.18571429 0.2 0.21428571 0.22857143 0.24285714 0.25714286 0.27142857 0.28571429 0.3 0.31428571 0.32857143 0.34285714 0.35714286 0.37142857 0.38571429 0.4 0.41428571 0.42857143 0.44285714 0.45714286 0.47142857 0.48571429 0.5 0.51428571 0.52857143 0.54285714 0.55714286 0.57142857 0.58571429 0.6 0.61428571 0.62857143 0.64285714 0.65714286 0.67142857 0.68571429 0.7 0.71428571 0.72857143 0.74285714 0.75714286 0.77142857 0.78571429 0.8 0.81428571 0.82857143 0.84285714 0.85714286 0.87142857 0.88571429 0.9 0.91428571 0.92857143 0.94285714 0.95714286 0.97142857 0.98571429 1 1 1 1 1 1
  arc A9 (0.3577, 12.9951) -> (-0.3577, 12.9951) centre (0, 0) ccw
  spline S9 degree 5 poles (-0.9051, 11.2399) (-0.9055, 11.2449) (-0.9062, 11.255) (-0.9068, 11.27) (-0.907, 11.2901) (-0.9062, 11.3152) (-0.9047, 11.3404) (-0.9028, 11.3655) (-0.9006, 11.3907) (-0.8982, 11.416) (-0.8957, 11.4412) (-0.8929, 11.4664) (-0.8899, 11.4917) (-0.8866, 11.5169) (-0.8828, 11.5422) (-0.8788, 11.5674) (-0.8745, 11.5927) (-0.87, 11.6179) (-0.8652, 11.6432) (-0.8603, 11.6685) (-0.8552, 11.6937) (-0.8499, 11.719) (-0.8443, 11.7443) (-0.8386, 11.7695) (-0.8327, 11.7948) (-0.8265, 11.82) (-0.8202, 11.8453) (-0.8136, 11.8706) (-0.8069, 11.8958) (-0.8, 11.921) (-0.7929, 11.9463) (-0.7857, 11.9715) (-0.7783, 11.9967) (-0.7707, 12.0219) (-0.7629, 12.0471) (-0.755, 12.0723) (-0.7469, 12.0975) (-0.7387, 12.1227) (-0.7302, 12.1479) (-0.7217, 12.173) (-0.7129, 12.1982) (-0.7041, 12.2233) (-0.695, 12.2484) (-0.6858, 12.2735) (-0.6765, 12.2986) (-0.667, 12.3237) (-0.6573, 12.3488) (-0.6475, 12.3739) (-0.6376, 12.3989) (-0.6275, 12.424) (-0.6173, 12.449) (-0.6069, 12.474) (-0.5964, 12.499) (-0.5858, 12.5239) (-0.575, 12.5489) (-0.564, 12.5738) (-0.553, 12.5988) (-0.5418, 12.6237) (-0.5304, 12.6486) (-0.5189, 12.6735) (-0.5073, 12.6983) (-0.4956, 12.7232) (-0.4837, 12.748) (-0.4717, 12.7728) (-0.4595, 12.7976) (-0.4473, 12.8223) (-0.4349, 12.8471) (-0.4223, 12.8718) (-0.4097, 12.8965) (-0.3969, 12.9212) (-0.384, 12.9458) (-0.3735, 12.9655) (-0.3657, 12.9803) (-0.3604, 12.9902) (-0.3577, 12.9951) knots 0 0 0 0 0 0 0.01428571 0.02857143 0.04285714 0.05714286 0.07142857 0.08571429 0.1 0.11428571 0.12857143 0.14285714 0.15714286 0.17142857 0.18571429 0.2 0.21428571 0.22857143 0.24285714 0.25714286 0.27142857 0.28571429 0.3 0.31428571 0.32857143 0.34285714 0.35714286 0.37142857 0.38571429 0.4 0.41428571 0.42857143 0.44285714 0.45714286 0.47142857 0.48571429 0.5 0.51428571 0.52857143 0.54285714 0.55714286 0.57142857 0.58571429 0.6 0.61428571 0.62857143 0.64285714 0.65714286 0.67142857 0.68571429 0.7 0.71428571 0.72857143 0.74285714 0.75714286 0.77142857 0.78571429 0.8 0.81428571 0.82857143 0.84285714 0.85714286 0.87142857 0.88571429 0.9 0.91428571 0.92857143 0.94285714 0.95714286 0.97142857 0.98571429 1 1 1 1 1 1
  line L9 (-0.9051, 11.2399) -> (-0.8636, 10.7145)
  arc A10 (-0.8636, 10.7145) -> (-1.9389, 10.5729) centre (0, 0) ccw
  line L10 (-1.9389, 10.5729) -> (-2.0348, 11.0912)
  spline S10 degree 5 poles (-2.0348, 11.0912) (-2.0357, 11.0961) (-2.0377, 11.106) (-2.041, 11.1207) (-2.046, 11.1401) (-2.0533, 11.1642) (-2.0612, 11.1881) (-2.0696, 11.2119) (-2.0783, 11.2357) (-2.0871, 11.2594) (-2.096, 11.2831) (-2.1052, 11.3068) (-2.1147, 11.3304) (-2.1244, 11.3539) (-2.1346, 11.3774) (-2.145, 11.4007) (-2.1557, 11.424) (-2.1666, 11.4472) (-2.1777, 11.4704) (-2.189, 11.4935) (-2.2005, 11.5166) (-2.2122, 11.5397) (-2.2241, 11.5626) (-2.2361, 11.5855) (-2.2484, 11.6084) (-2.2609, 11.6312) (-2.2736, 11.654) (-2.2864, 11.6767) (-2.2995, 11.6993) (-2.3126, 11.7219) (-2.326, 11.7444) (-2.3395, 11.7669) (-2.3532, 11.7894) (-2.3671, 11.8118) (-2.3811, 11.8341) (-2.3953, 11.8564) (-2.4096, 11.8786) (-2.4241, 11.9008) (-2.4387, 11.9229) (-2.4535, 11.945) (-2.4685, 11.967) (-2.4836, 11.989) (-2.4988, 12.011) (-2.5142, 12.0328) (-2.5297, 12.0547) (-2.5454, 12.0764) (-2.5612, 12.0982) (-2.5771, 12.1198) (-2.5932, 12.1415) (-2.6094, 12.163) (-2.6258, 12.1846) (-2.6423, 12.206) (-2.6589, 12.2274) (-2.6756, 12.2488) (-2.6925, 12.2701) (-2.7095, 12.2914) (-2.7267, 12.3126) (-2.744, 12.3338) (-2.7614, 12.3549) (-2.7789, 12.3759) (-2.7965, 12.3969) (-2.8143, 12.4179) (-2.8322, 12.4388) (-2.8502, 12.4596) (-2.8684, 12.4804) (-2.8866, 12.5012) (-2.905, 12.5219) (-2.9235, 12.5425) (-2.9421, 12.5631) (-2.9609, 12.5836) (-2.9797, 12.6041) (-2.9949, 12.6204) (-3.0064, 12.6327) (-3.014, 12.6408) (-3.0178, 12.6449) knots 0 0 0 0 0 0 0.01428571 0.02857143 0.04285714 0.05714286 0.07142857 0.08571429 0.1 0.11428571 0.12857143 0.14285714 0.15714286 0.17142857 0.18571429 0.2 0.21428571 0.22857143 0.24285714 0.25714286 0.27142857 0.28571429 0.3 0.31428571 0.32857143 0.34285714 0.35714286 0.37142857 0.38571429 0.4 0.41428571 0.42857143 0.44285714 0.45714286 0.47142857 0.48571429 0.5 0.51428571 0.52857143 0.54285714 0.55714286 0.57142857 0.58571429 0.6 0.61428571 0.62857143 0.64285714 0.65714286 0.67142857 0.68571429 0.7 0.71428571 0.72857143 0.74285714 0.75714286 0.77142857 0.78571429 0.8 0.81428571 0.82857143 0.84285714 0.85714286 0.87142857 0.88571429 0.9 0.91428571 0.92857143 0.94285714 0.95714286 0.97142857 0.98571429 1 1 1 1 1 1
  arc A11 (-3.0178, 12.6449) -> (-3.7089, 12.4597) centre (0, 0) ccw
  spline S11 degree 5 poles (-3.7834, 10.6227) (-3.7851, 10.6274) (-3.7883, 10.6369) (-3.7928, 10.6513) (-3.7981, 10.6706) (-3.8039, 10.6951) (-3.809, 10.7198) (-3.8136, 10.7446) (-3.818, 10.7695) (-3.8223, 10.7945) (-3.8264, 10.8195) (-3.8302, 10.8446) (-3.8339, 10.8698) (-3.8371, 10.895) (-3.8401, 10.9204) (-3.8427, 10.9458) (-3.8451, 10.9713) (-3.8473, 10.9969) (-3.8492, 11.0225) (-3.851, 11.0482) (-3.8526, 11.0739) (-3.854, 11.0997) (-3.8552, 11.1256) (-3.8562, 11.1514) (-3.857, 11.1774) (-3.8576, 11.2034) (-3.858, 11.2294) (-3.8582, 11.2555) (-3.8583, 11.2816) (-3.8581, 11.3078) (-3.8578, 11.334) (-3.8574, 11.3602) (-3.8567, 11.3865) (-3.8559, 11.4128) (-3.855, 11.4392) (-3.8538, 11.4656) (-3.8525, 11.492) (-3.8511, 11.5184) (-3.8495, 11.5449) (-3.8477, 11.5714) (-3.8458, 11.598) (-3.8437, 11.6246) (-3.8415, 11.6512) (-3.8391, 11.6778) (-3.8365, 11.7045) (-3.8339, 11.7312) (-3.831, 11.7579) (-3.8281, 11.7846) (-3.825, 11.8114) (-3.8217, 11.8382) (-3.8183, 11.865) (-3.8147, 11.8919) (-3.8111, 11.9187) (-3.8072, 11.9456) (-3.8033, 11.9725) (-3.7992, 11.9994) (-3.7949, 12.0264) (-3.7905, 12.0533) (-3.786, 12.0803) (-3.7814, 12.1073) (-3.7766, 12.1343) (-3.7717, 12.1614) (-3.7666, 12.1884) (-3.7614, 12.2155) (-3.7561, 12.2426) (-3.7507, 12.2696) (-3.7451, 12.2968) (-3.7394, 12.3239) (-3.7336, 12.351) (-3.7276, 12.3782) (-3.7215, 12.4053) (-3.7165, 12.4271) (-3.7127, 12.4434) (-3.7102, 12.4543) (-3.7089, 12.4597) knots 0 0 0 0 0 0 0.01428571 0.02857143 0.04285714 0.05714286 0.07142857 0.08571429 0.1 0.11428571 0.12857143 0.14285714 0.15714286 0.17142857 0.18571429 0.2 0.21428571 0.22857143 0.24285714 0.25714286 0.27142857 0.28571429 0.3 0.31428571 0.32857143 0.34285714 0.35714286 0.37142857 0.38571429 0.4 0.41428571 0.42857143 0.44285714 0.45714286 0.47142857 0.48571429 0.5 0.51428571 0.52857143 0.54285714 0.55714286 0.57142857 0.58571429 0.6 0.61428571 0.62857143 0.64285714 0.65714286 0.67142857 0.68571429 0.7 0.71428571 0.72857143 0.74285714 0.75714286 0.77142857 0.78571429 0.8 0.81428571 0.82857143 0.84285714 0.85714286 0.87142857 0.88571429 0.9 0.91428571 0.92857143 0.94285714 0.95714286 0.97142857 0.98571429 1 1 1 1 1 1
  line L11 (-3.7834, 10.6227) -> (-3.6073, 10.1259)
  arc A12 (-3.6073, 10.1259) -> (-4.6093, 9.7108) centre (0, 0) ccw
  line L12 (-4.6093, 9.7108) -> (-4.8361, 10.1866)
  spline S12 degree 5 poles (-4.8361, 10.1866) (-4.8383, 10.1912) (-4.8427, 10.2002) (-4.8497, 10.2135) (-4.8596, 10.231) (-4.8728, 10.2523) (-4.8867, 10.2734) (-4.901, 10.2942) (-4.9155, 10.315) (-4.9301, 10.3356) (-4.9449, 10.3562) (-4.9599, 10.3767) (-4.9751, 10.397) (-4.9907, 10.4172) (-5.0065, 10.4372) (-5.0226, 10.4571) (-5.039, 10.4768) (-5.0555, 10.4964) (-5.0723, 10.5159) (-5.0892, 10.5353) (-5.1063, 10.5547) (-5.1235, 10.5739) (-5.1409, 10.593) (-5.1585, 10.612) (-5.1763, 10.6309) (-5.1942, 10.6497) (-5.2124, 10.6684) (-5.2307, 10.687) (-5.2491, 10.7055) (-5.2677, 10.7239) (-5.2864, 10.7422) (-5.3053, 10.7605) (-5.3243, 10.7786) (-5.3435, 10.7966) (-5.3628, 10.8146) (-5.3823, 10.8324) (-5.4019, 10.8502) (-5.4216, 10.8679) (-5.4415, 10.8855) (-5.4615, 10.903) (-5.4817, 10.9204) (-5.5019, 10.9377) (-5.5223, 10.955) (-5.5428, 10.9721) (-5.5635, 10.9892) (-5.5842, 11.0062) (-5.6051, 11.023) (-5.6261, 11.0399) (-5.6473, 11.0566) (-5.6685, 11.0732) (-5.6899, 11.0898) (-5.7114, 11.1062) (-5.733, 11.1226) (-5.7547, 11.1389) (-5.7765, 11.1552) (-5.7985, 11.1713) (-5.8205, 11.1873) (-5.8427, 11.2033) (-5.8649, 11.2192) (-5.8873, 11.235) (-5.9098, 11.2507) (-5.9324, 11.2664) (-5.9551, 11.2819) (-5.9779, 11.2974) (-6.0008, 11.3128) (-6.0238, 11.3281) (-6.0469, 11.3433) (-6.0701, 11.3585) (-6.0935, 11.3735) (-6.1169, 11.3885) (-6.1404, 11.4034) (-6.1593, 11.4153) (-6.1735, 11.4241) (-6.183, 11.43) (-6.1877, 11.4329) knots 0 0 0 0 0 0 0.01428571 0.02857143 0.04285714 0.05714286 0.07142857 0.08571429 0.1 0.11428571 0.12857143 0.14285714 0.15714286 0.17142857 0.18571429 0.2 0.21428571 0.22857143 0.24285714 0.25714286 0.27142857 0.28571429 0.3 0.31428571 0.32857143 0.34285714 0.35714286 0.37142857 0.38571429 0.4 0.41428571 0.42857143 0.44285714 0.45714286 0.47142857 0.48571429 0.5 0.51428571 0.52857143 0.54285714 0.55714286 0.57142857 0.58571429 0.6 0.61428571 0.62857143 0.64285714 0.65714286 0.67142857 0.68571429 0.7 0.71428571 0.72857143 0.74285714 0.75714286 0.77142857 0.78571429 0.8 0.81428571 0.82857143 0.84285714 0.85714286 0.87142857 0.88571429 0.9 0.91428571 0.92857143 0.94285714 0.95714286 0.97142857 0.98571429 1 1 1 1 1 1
  arc A13 (-6.1877, 11.4329) -> (-6.8073, 11.0752) centre (0, 0) ccw
  spline S13 degree 5 poles (-6.4038, 9.2815) (-6.4067, 9.2856) (-6.4123, 9.294) (-6.4203, 9.3067) (-6.4305, 9.324) (-6.4424, 9.3462) (-6.4537, 9.3687) (-6.4646, 9.3915) (-6.4753, 9.4144) (-6.4859, 9.4374) (-6.4963, 9.4605) (-6.5065, 9.4837) (-6.5165, 9.5071) (-6.5262, 9.5307) (-6.5356, 9.5544) (-6.5448, 9.5783) (-6.5537, 9.6023) (-6.5624, 9.6264) (-6.5709, 9.6507) (-6.5793, 9.675) (-6.5875, 9.6995) (-6.5955, 9.724) (-6.6034, 9.7487) (-6.611, 9.7734) (-6.6185, 9.7983) (-6.6258, 9.8232) (-6.6329, 9.8483) (-6.6399, 9.8734) (-6.6467, 9.8986) (-6.6533, 9.9239) (-6.6598, 9.9493) (-6.6662, 9.9748) (-6.6724, 10.0003) (-6.6784, 10.0259) (-6.6843, 10.0516) (-6.69, 10.0774) (-6.6956, 10.1033) (-6.701, 10.1292) (-6.7063, 10.1552) (-6.7115, 10.1813) (-6.7165, 10.2074) (-6.7214, 10.2337) (-6.7261, 10.2599) (-6.7307, 10.2863) (-6.7352, 10.3127) (-6.7395, 10.3392) (-6.7437, 10.3657) (-6.7477, 10.3923) (-6.7516, 10.419) (-6.7554, 10.4457) (-6.7591, 10.4725) (-6.7626, 10.4993) (-6.766, 10.5262) (-6.7693, 10.5532) (-6.7724, 10.5802) (-6.7754, 10.6073) (-6.7783, 10.6344) (-6.781, 10.6616) (-6.7836, 10.6888) (-6.7861, 10.7161) (-6.7885, 10.7434) (-6.7908, 10.7708) (-6.7929, 10.7982) (-6.7949, 10.8257) (-6.7967, 10.8532) (-6.7985, 10.8808) (-6.8001, 10.9085) (-6.8016, 10.9361) (-6.803, 10.9638) (-6.8043, 10.9916) (-6.8054, 11.0194) (-6.8063, 11.0417) (-6.8068, 11.0585) (-6.8072, 11.0696) (-6.8073, 11.0752) knots 0 0 0 0 0 0 0.01428571 0.02857143 0.04285714 0.05714286 0.07142857 0.08571429 0.1 0.11428571 0.12857143 0.14285714 0.15714286 0.17142857 0.18571429 0.2 0.21428571 0.22857143 0.24285714 0.25714286 0.27142857 0.28571429 0.3 0.31428571 0.32857143 0.34285714 0.35714286 0.37142857 0.38571429 0.4 0.41428571 0.42857143 0.44285714 0.45714286 0.47142857 0.48571429 0.5 0.51428571 0.52857143 0.54285714 0.55714286 0.57142857 0.58571429 0.6 0.61428571 0.62857143 0.64285714 0.65714286 0.67142857 0.68571429 0.7 0.71428571 0.72857143 0.74285714 0.75714286 0.77142857 0.78571429 0.8 0.81428571 0.82857143 0.84285714 0.85714286 0.87142857 0.88571429 0.9 0.91428571 0.92857143 0.94285714 0.95714286 0.97142857 0.98571429 1 1 1 1 1 1
  line L13 (-6.4038, 9.2815) -> (-6.1051, 8.8472)
  arc A14 (-6.1051, 8.8472) -> (-6.9656, 8.1869) centre (0, 0) ccw
  line L14 (-6.9656, 8.1869) -> (-7.3078, 8.5878)
  spline S14 degree 5 poles (-7.3078, 8.5878) (-7.3111, 8.5917) (-7.3177, 8.5992) (-7.3279, 8.6103) (-7.342, 8.6246) (-7.3603, 8.6418) (-7.3791, 8.6586) (-7.3983, 8.675) (-7.4177, 8.6913) (-7.4372, 8.7074) (-7.4568, 8.7235) (-7.4766, 8.7394) (-7.4966, 8.7551) (-7.5168, 8.7706) (-7.5373, 8.7858) (-7.558, 8.8008) (-7.5789, 8.8156) (-7.6, 8.8303) (-7.6212, 8.8448) (-7.6425, 8.8592) (-7.664, 8.8734) (-7.6856, 8.8875) (-7.7074, 8.9015) (-7.7293, 8.9153) (-7.7514, 8.929) (-7.7736, 8.9425) (-7.796, 8.9558) (-7.8184, 8.9691) (-7.841, 8.9822) (-7.8638, 8.9951) (-7.8866, 9.008) (-7.9096, 9.0207) (-7.9326, 9.0333) (-7.9558, 9.0457) (-7.9791, 9.0581) (-8.0025, 9.0703) (-8.0261, 9.0824) (-8.0497, 9.0943) (-8.0735, 9.1062) (-8.0973, 9.1179) (-8.1213, 9.1295) (-8.1453, 9.141) (-8.1695, 9.1524) (-8.1938, 9.1637) (-8.2181, 9.1748) (-8.2426, 9.1858) (-8.2671, 9.1967) (-8.2918, 9.2075) (-8.3165, 9.2182) (-8.3413, 9.2288) (-8.3663, 9.2392) (-8.3913, 9.2496) (-8.4164, 9.2598) (-8.4416, 9.27) (-8.4669, 9.28) (-8.4922, 9.2899) (-8.5177, 9.2997) (-8.5432, 9.3094) (-8.5688, 9.319) (-8.5945, 9.3284) (-8.6203, 9.3378) (-8.6462, 9.347) (-8.6722, 9.3562) (-8.6982, 9.3652) (-8.7243, 9.3742) (-8.7505, 9.383) (-8.7768, 9.3917) (-8.8031, 9.4004) (-8.8295, 9.4089) (-8.856, 9.4173) (-8.8826, 9.4256) (-8.9039, 9.4321) (-8.9199, 9.437) (-8.9306, 9.4403) (-8.936, 9.4419) knots 0 0 0 0 0 0 0.01428571 0.02857143 0.04285714 0.05714286 0.07142857 0.08571429 0.1 0.11428571 0.12857143 0.14285714 0.15714286 0.17142857 0.18571429 0.2 0.21428571 0.22857143 0.24285714 0.25714286 0.27142857 0.28571429 0.3 0.31428571 0.32857143 0.34285714 0.35714286 0.37142857 0.38571429 0.4 0.41428571 0.42857143 0.44285714 0.45714286 0.47142857 0.48571429 0.5 0.51428571 0.52857143 0.54285714 0.55714286 0.57142857 0.58571429 0.6 0.61428571 0.62857143 0.64285714 0.65714286 0.67142857 0.68571429 0.7 0.71428571 0.72857143 0.74285714 0.75714286 0.77142857 0.78571429 0.8 0.81428571 0.82857143 0.84285714 0.85714286 0.87142857 0.88571429 0.9 0.91428571 0.92857143 0.94285714 0.95714286 0.97142857 0.98571429 1 1 1 1 1 1
  arc A15 (-8.936, 9.4419) -> (-9.4419, 8.936) centre (0, 0) ccw
  spline S15 degree 5 poles (-8.5878, 7.3078) (-8.5917, 7.3111) (-8.5992, 7.3177) (-8.6103, 7.3279) (-8.6246, 7.342) (-8.6418, 7.3603) (-8.6586, 7.3791) (-8.675, 7.3983) (-8.6913, 7.4177) (-8.7074, 7.4372) (-8.7235, 7.4568) (-8.7394, 7.4766) (-8.7551, 7.4966) (-8.7706, 7.5168) (-8.7858, 7.5373) (-8.8008, 7.558) (-8.8156, 7.5789) (-8.8303, 7.6) (-8.8448, 7.6212) (-8.8592, 7.6425) (-8.8734, 7.664) (-8.8875, 7.6856) (-8.9015, 7.7074) (-8.9153, 7.7293) (-8.929, 7.7514) (-8.9425, 7.7736) (-8.9558, 7.796) (-8.9691, 7.8184) (-8.9822, 7.841) (-8.9951, 7.8638) (-9.008, 7.8866) (-9.0207, 7.9096) (-9.0333, 7.9326) (-9.0457, 7.9558) (-9.0581, 7.9791) (-9.0703, 8.0025) (-9.0824, 8.0261) (-9.0943, 8.0497) (-9.1062, 8.0735) (-9.1179, 8.0973) (-9.1295, 8.1213) (-9.141, 8.1453) (-9.1524, 8.1695) (-9.1637, 8.1938) (-9.1748, 8.2181) (-9.1858, 8.2426) (-9.1967, 8.2671) (-9.2075, 8.2918) (-9.2182, 8.3165) (-9.2288, 8.3413) (-9.2392, 8.3663) (-9.2496, 8.3913) (-9.2598, 8.4164) (-9.27, 8.4416) (-9.28, 8.4669) (-9.2899, 8.4922) (-9.2997, 8.5177) (-9.3094, 8.5432) (-9.319, 8.5688) (-9.3284, 8.5945) (-9.3378, 8.6203) (-9.347, 8.6462) (-9.3562, 8.6722) (-9.3652, 8.6982) (-9.3742, 8.7243) (-9.383, 8.7505) (-9.3917, 8.7768) (-9.4004, 8.8031) (-9.4089, 8.8295) (-9.4173, 8.856) (-9.4256, 8.8826) (-9.4321, 8.9039) (-9.437, 8.9199) (-9.4403, 8.9306) (-9.4419, 8.936) knots 0 0 0 0 0 0 0.01428571 0.02857143 0.04285714 0.05714286 0.07142857 0.08571429 0.1 0.11428571 0.12857143 0.14285714 0.15714286 0.17142857 0.18571429 0.2 0.21428571 0.22857143 0.24285714 0.25714286 0.27142857 0.28571429 0.3 0.31428571 0.32857143 0.34285714 0.35714286 0.37142857 0.38571429 0.4 0.41428571 0.42857143 0.44285714 0.45714286 0.47142857 0.48571429 0.5 0.51428571 0.52857143 0.54285714 0.55714286 0.57142857 0.58571429 0.6 0.61428571 0.62857143 0.64285714 0.65714286 0.67142857 0.68571429 0.7 0.71428571 0.72857143 0.74285714 0.75714286 0.77142857 0.78571429 0.8 0.81428571 0.82857143 0.84285714 0.85714286 0.87142857 0.88571429 0.9 0.91428571 0.92857143 0.94285714 0.95714286 0.97142857 0.98571429 1 1 1 1 1 1
  line L15 (-8.5878, 7.3078) -> (-8.1869, 6.9656)
  arc A16 (-8.1869, 6.9656) -> (-8.8472, 6.1051) centre (0, 0) ccw
  line L16 (-8.8472, 6.1051) -> (-9.2815, 6.4038)